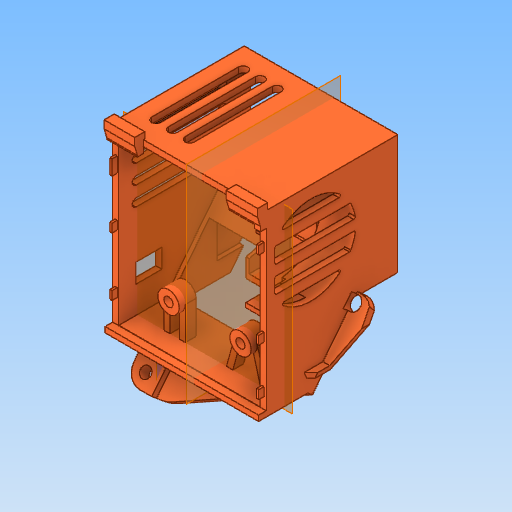
# Autodesk Inventor part: кожух2
Saved by Autodesk Inventor 2017 (Build 210142000, 142)
## iProperties
Part Number: кожух2
Material: Типовые
Document SubType Name: Modeling
Designer: Max
Mass: 19.7684 g
Surface Area: 231.932 cm^2
Volume: 19.7684 cm^3
Density: 1 g/cm^3
Appearance: Оранжевый
Author: Max
Autodesk Inventor part; units mm, degrees
ref_plane "YZ Plane" through (0, 0, 0) normal (1, 0, 0) x (0, 1, 0)
ref_plane "XZ Plane" through (0, 0, 0) normal (0, 1, 0) x (-1, 0, 0)
ref_plane "XY Plane" through (0, 0, 0) normal (0, 0, 1) x (1, 0, 0)
sketch "Эскиз1" plane through (0, 0, 0) normal (0, 0, 1) x (1, 0, 0)
  line L0 (1.3628, -26.8991) -> (1.3628, -29.3491) projected
  line L1 (1.3628, -29.3491) -> (24.1628, -29.3491) projected
  line L2 (24.1628, -29.3491) -> (24.1628, -4.9691) projected
  line L3 (24.1628, -4.9691) -> (13.8628, -4.9691) projected
  line L4 (13.8628, -4.9691) -> (13.8628, 12.3409) projected
  line L5 (13.8628, 12.3409) -> (24.1628, 12.3409) projected
  line L6 (24.1628, 12.3409) -> (24.1628, 22.1409) projected
  line L7 (24.1628, 22.1409) -> (22.1628, 22.1409) projected
  line L8 (22.1628, 22.1409) -> (22.1628, 23.2409) projected
  line L9 (22.1628, 23.2409) -> (19.7628, 23.2409) projected
  line L10 (19.7628, 23.2409) -> (19.7628, 20.2409) projected
  line L11 (19.7628, 20.2409) -> (15.3628, 20.2409) projected
  line L12 (15.3628, 20.2409) -> (15.3628, 23.2409) projected
  line L13 (15.3628, 23.2409) -> (13.8628, 23.2409) projected
  line L14 (13.8628, 23.2409) -> (13.8628, 27.2009) projected
  line L15 (13.8628, 27.2009) -> (-16.0172, 27.2009) projected
  line L16 (-16.0172, 27.2009) -> (-16.0172, 23.2409) projected
  line L17 (-16.0172, 23.2409) -> (-17.1172, 23.2409) projected
  line L18 (-17.1172, 23.2409) -> (-17.1172, 20.2009) projected
  line L19 (-17.1172, 20.2009) -> (-21.5172, 20.2009) projected
  line L20 (-21.5172, 20.2009) -> (-21.5172, 23.2409) projected
  line L21 (-21.5172, 23.2409) -> (-26.0172, 23.2409) projected
  line L22 (-26.0172, 23.2409) -> (-26.0172, -29.3491) projected
  line L23 (-26.0172, -29.3491) -> (-3.1372, -29.3491) projected
  line L24 (-3.1372, -29.3491) -> (-3.1372, -26.8991) projected
  line L25 (-3.1372, -26.8991) -> (1.3628, -26.8991) projected
  line L26 (-6.6027, 20.9009) -> (-7.4672, 20.9009) projected
  arc A0 (-6.6027, 20.9009) -> (-7.2289, 20.2627) centre (-4.7984, 18.5041) ccw projected
  line L27 (-7.2289, 20.2627) -> (-8.0672, 19.1042) projected
  arc A1 (-5.6572, 17.7284) -> (-8.0672, 19.1042) centre (-12.3972, 8.7209) ccw projected
  line L28 (-5.6572, 17.7284) -> (0.0428, 23.0709) projected
  line L29 (0.0428, 23.0709) -> (1.0428, 23.0709) projected
  line L30 (1.0428, 23.0709) -> (1.0428, -5.6291) projected
  line L31 (1.0428, -5.6291) -> (0.0428, -5.6291) projected
  line L32 (0.0428, -5.6291) -> (-3.9933, -1.8461) projected
  arc A2 (-3.9933, -1.8461) -> (-7.3822, -1.3495) centre (-6.0449, -4.0349) ccw projected
  arc A3 (-14.1715, 19.8301) -> (-7.3822, -1.3495) centre (-12.3972, 8.7209) ccw projected
  line L33 (-14.1715, 19.8301) -> (-7.4672, 20.9009) projected
  line L34 (3.2328, 20.0509) -> (3.2328, 26.3009) projected
  line L35 (3.2328, 26.3009) -> (11.7328, 26.3009) projected
  line L36 (11.7328, 26.3009) -> (11.7328, 20.0509) projected
  line L37 (11.7328, 20.0509) -> (3.2328, 20.0509) projected
  line L38 (2.9428, -9.0491) -> (2.9428, -2.8491) projected
  line L39 (2.9428, -2.8491) -> (11.3928, -2.8491) projected
  line L40 (11.3928, -2.8491) -> (11.3928, -9.0491) projected
  line L41 (11.3928, -9.0491) -> (2.9428, -9.0491) projected
  line L42 (11.1828, 15.3909) -> (11.1828, 4.1309) projected
  line L43 (11.1828, 4.1309) -> (3.5128, 4.1309) projected
  line L44 (3.5128, 4.1309) -> (3.5128, 15.3909) projected
  line L45 (3.5128, 15.3909) -> (5.2778, 15.3909) projected
  line L46 (5.2778, 15.3909) -> (5.2778, 7.1309) projected
  line L47 (5.2778, 7.1309) -> (9.4178, 7.1309) projected
  line L48 (9.4178, 7.1309) -> (9.4178, 15.3909) projected
  line L49 (9.4178, 15.3909) -> (11.1828, 15.3909) projected
  line L50 (-16.0372, -26.1691) -> (-16.0372, -22.6691) projected
  line L51 (-16.0372, -22.6691) -> (-10.7672, -22.6691) projected
  line L52 (-10.7672, -22.6691) -> (-10.7672, -26.1691) projected
  line L53 (-10.7672, -26.1691) -> (-16.0372, -26.1691) projected
  line L54 (-21.1172, -9.1491) -> (-21.1172, -6.5491) projected
  line L55 (-21.1172, -6.5491) -> (-15.8172, -6.5491) projected
  line L56 (-15.8172, -6.5491) -> (-15.8172, -9.1491) projected
  line L57 (-15.8172, -9.1491) -> (-21.1172, -9.1491) projected
  circle A4 centre (16.8328, -11.1491) radius 2.05 projected
  circle A5 centre (-11.7672, -18.4991) radius 2.05 projected
  circle A6 centre (11.7328, -18.4991) radius 2.05 projected
  circle A7 centre (-1.1672, -11.1291) radius 1.9 projected
  circle A8 centre (17.9828, 16.4009) radius 1.15 projected
  line L58 (-25.2172, 13.4509) -> (-25.2172, 18.3509) projected
  line L59 (-25.2172, 18.3509) -> (-24.5172, 18.3509) projected
  line L60 (-24.5172, 18.3509) -> (-24.5172, 13.4509) projected
  line L61 (-24.5172, 13.4509) -> (-25.2172, 13.4509) projected
  line L62 (-25.2172, -2.6491) -> (-25.2172, 0.1509) projected
  line L63 (-25.2172, 0.1509) -> (-24.5172, 0.1509) projected
  line L64 (-24.5172, 0.1509) -> (-24.5172, -2.6491) projected
  line L65 (-24.5172, -2.6491) -> (-25.2172, -2.6491) projected
  line L66 (-25.2172, -21.7291) -> (-25.2172, -18.9291) projected
  line L67 (-25.2172, -18.9291) -> (-24.5172, -18.9291) projected
  line L68 (-24.5172, -18.9291) -> (-24.5172, -21.7291) projected
  line L69 (-24.5172, -21.7291) -> (-25.2172, -21.7291) projected
  line L70 (22.7628, 15.1009) -> (22.7628, 17.9009) projected
  line L71 (22.7628, 17.9009) -> (23.4628, 17.9009) projected
  line L72 (23.4628, 17.9009) -> (23.4628, 15.1009) projected
  line L73 (23.4628, 15.1009) -> (22.7628, 15.1009) projected
  line L74 (22.7628, -25.7691) -> (22.7628, -22.9691) projected
  line L75 (22.7628, -22.9691) -> (23.4628, -22.9691) projected
  line L76 (23.4628, -22.9691) -> (23.4628, -25.7691) projected
  line L77 (23.4628, -25.7691) -> (22.7628, -25.7691) projected
  line L78 (22.7628, -10.3691) -> (22.7628, -7.5691) projected
  line L79 (22.7628, -7.5691) -> (23.4628, -7.5691) projected
  line L80 (23.4628, -7.5691) -> (23.4628, -10.3691) projected
  line L81 (23.4628, -10.3691) -> (22.7628, -10.3691) projected
  line L82 (-26.0172, -31.2191) -> (24.1628, -31.2191)
  line L83 (24.1628, -31.2191) -> (24.1628, 27.2009)
  line L84 (24.1628, 27.2009) -> (-26.0172, 27.2009)
  line L85 (-26.0172, 29.2009) -> (-26.0172, -31.2191)
  line L86 (-26.0172, -29.3491) -> (24.1628, -29.3491)
  line L87 (-24.0172, -29.3491) -> (-24.0172, 23.2409)
  line L88 (22.1628, -29.3491) -> (22.1628, 23.2409)
  line L89 (-16.0172, 23.2409) -> (-26.0172, 23.2409)
  line L90 (-26.0172, 29.2009) -> (-16.0172, 29.2009)
  line L91 (-16.0172, 29.2009) -> (-16.0172, 23.2409)
  line L92 (13.8628, 23.2409) -> (22.1628, 23.2409)
  line L93 (24.1628, 23.2409) -> (24.1628, 29.2009)
  line L94 (24.1628, 29.2009) -> (13.8628, 29.2009)
  line L95 (13.8628, 29.2009) -> (13.8628, 23.2409)
  line L96 (22.1628, 22.1409) -> (24.1628, 22.1409)
  line L97 (-26.0172, 23.2409) -> (-26.0172, 29.2009)
  line L98 (-26.0172, -31.2191) -> (24.1628, -31.2191)
  line L99 (24.1628, -31.2191) -> (24.1628, -29.3491)
  line L100 (24.1628, -29.3491) -> (-26.0172, -29.3491)
  line L101 (-26.0172, -29.3491) -> (-26.0172, -31.2191)
  line L102 (22.1628, 22.1409) -> (24.1628, 22.1409)
  line L103 (24.1628, 22.1409) -> (24.1628, -29.3491)
  line L104 (24.1628, -29.3491) -> (22.1628, -29.3491)
  line L105 (22.1628, -29.3491) -> (22.1628, 22.1409)
  line L106 (-24.0172, 23.2409) -> (-26.0172, 23.2409)
  line L107 (-26.0172, 23.2409) -> (-26.0172, -29.3491)
  line L108 (-26.0172, -29.3491) -> (-24.0172, -29.3491)
  line L109 (-24.0172, -29.3491) -> (-24.0172, 23.2409)
  line L110 (-16.0172, 27.2009) -> (13.8628, 27.2009)
  line L111 (13.8628, 27.2009) -> (13.8628, 25.2009)
  line L112 (24.1628, 25.2009) -> (-26.0172, 25.2009)
  line L113 (-16.0172, 25.2009) -> (-16.0172, 27.2009)
  line L114 (24.1628, 25.2009) -> (13.8628, 25.2009)
  line L115 (13.8628, 25.2009) -> (13.8628, 27.2009)
  line L116 (13.8628, 27.2009) -> (24.1628, 27.2009)
  line L117 (24.1628, 27.2009) -> (24.1628, 25.2009)
  line L118 (-26.0172, 25.2009) -> (-16.0172, 25.2009)
  line L119 (-16.0172, 25.2009) -> (-16.0172, 27.2009)
  line L120 (-16.0172, 27.2009) -> (-26.0172, 27.2009)
  line L121 (-26.0172, 27.2009) -> (-26.0172, 25.2009)
  line L122 (-24.0172, 23.2409) -> (-26.0172, 23.2409)
  line L123 (-26.0172, 23.2409) -> (-26.0172, 25.2009)
  line L124 (-26.0172, 25.2009) -> (-24.0172, 25.2009)
  line L125 (-24.0172, 25.2009) -> (-24.0172, 23.2409)
  line L126 (22.1628, 22.1409) -> (24.1628, 22.1409)
  line L127 (24.1628, 22.1409) -> (24.1628, 25.2009)
  line L128 (24.1628, 25.2009) -> (22.1628, 25.2009)
  line L129 (22.1628, 25.2009) -> (22.1628, 22.1409)
  point P0 (0, 0)
  dimension "d0" = 1.87
  dimension "d1" = 2
  dimension "d2" = 2
  dimension "d3" = 2
  dimension "d6" = 2
  constraints: 96 end point, 22 parallel, 13 point on line, 11 horizontal, 11 perpendicular, 7 collinear, 1 vertical
  measures "d0" distance between parallel lines of L23 L82
  measures "d1" distance between parallel lines of L87 L22
  measures "d2" distance between parallel lines of L83 L88
  measures "d3" distance between parallel lines of L15 L90
  measures "d6" distance between parallel lines of L15 L112
extrude "Выдавливание1" add sketch "Эскиз1" against normal blind 43 contours L1 L83 L82 L85 L23 L86 | L88 L3 L2 L1 | L88 L5 L83 L3 | L23 L22 L21 L87 | L88 L7 L6 L5 | L21 L85 L112 L125 | L8 L129 L112 L83 L7 | L112 L85 L84 L16 | L16 L15 L14 L112 L36 L35 L34 | L112 L14 L84 L83 | L85 L90 L91 L84 | L34 L35 L36 L112 | L58 L59 L60 L61 | L62 L63 L64 L65 | L66 L67 L68 L69 | L70 L71 L72 L73 | L74 L75 L76 L77 | L78 L79 L80 L81
extrude "Выдавливание2" cut sketch "Эскиз1" against normal blind 43 contours L85 L90 L91 L84
sketch "Эскиз2" plane through (0, 0, 0) normal (0, 0, 1) x (1, 0, 0)
  line L0 (-16.0172, 29.2009) -> (-16.0172, 23.2409) projected
  line L1 (-26.0172, 29.2009) -> (-16.0172, 29.2009) projected
  line L2 (-16.0172, 23.2409) -> (-26.0172, 23.2409) projected
  line L3 (13.8628, 23.2409) -> (13.8628, 27.2009) projected
  line L4 (13.8628, 29.2009) -> (13.8628, 23.2409) projected
  line L5 (24.1628, 29.2009) -> (13.8628, 29.2009) projected
  line L6 (24.1628, 23.2409) -> (24.1628, 29.2009) projected
  line L7 (24.1628, 22.1409) -> (22.1628, 22.1409) projected
  line L8 (22.1628, 25.2009) -> (22.1628, -29.3491) projected
  line L9 (22.1628, 23.2409) -> (19.7628, 23.2409) projected
  line L10 (13.8628, 23.2409) -> (22.1628, 23.2409) projected
  line L11 (24.1628, 23.2409) -> (24.1628, 22.1409)
  line L12 (24.1628, -31.2191) -> (24.1628, 27.2009) projected
  line L13 (-26.0172, 23.2409) -> (-26.0172, 29.2009)
  line L14 (-26.0172, -31.2191) -> (-26.0172, 27.2009) projected
  point P0 (0, 0)
  constraints: 4 end point, 2 collinear
extrude "Выдавливание3" add sketch "Эскиз2" along normal blind 2.8
sketch "Эскиз3" plane through (24.1628, -31.2191, -43) normal (1, 0, 0) x (0, 0, -1)
  line L0 (-43, 53.36) -> (-45.8, 53.36) projected
  line L1 (-44.92, 53.36) -> (-44.92, 54.8992)
  line L2 (-44.92, 54.8992) -> (-45.8, 57.8704)
  line L3 (-45.8, 53.36) -> (-45.8, 60.42) projected
  line L4 (-45.8, 54.46) -> (-45.8, 53.36) projected
  line L5 (-45.8, 57.8704) -> (-45.8, 53.36)
  line L6 (-44.92, 53.36) -> (-45.8, 53.36)
  point P0 (-43, 31.2191)
  dimension "d11" = 1.92
  constraints: 8 end point, 2 collinear, 2 point on line, 1 vertical
  measures "d11" distance from line of L0.start L1
extrude "Выдавливание4" cut sketch "Эскиз3" against normal blind 55
extrude "Выдавливание5" add sketch "Эскиз1" along normal blind 1.73 contours L58 L59 L60 L61 | L62 L63 L64 L65 | L66 L67 L68 L69 | L70 L71 L72 L73 | L74 L75 L76 L77 | L78 L79 L80 L81
sketch "Эскиз4" plane through (0, 0, 0) normal (0, 0, 1) x (1, 0, 0)
  line L0 (-26.0172, -31.2191) -> (24.1628, -31.2191) projected
  line L1 (-26.0172, -31.2191) -> (24.1628, -31.2191)
  line L2 (24.1628, -31.2191) -> (24.1628, -29.4423)
  line L3 (24.1628, -29.4423) -> (-26.0172, -29.4423)
  line L4 (-26.0172, -29.4423) -> (-26.0172, -31.2191)
  point P0 (0, 0)
  constraints: 8 end point, 2 parallel, 1 horizontal, 1 perpendicular
extrude "Выдавливание6" add sketch "Эскиз4" along normal blind 2.5
sketch "Эскиз5" plane through (24.1628, -31.2191, -43) normal (1, 0, 0) x (0, 0, -1)
  arc A0 (-42.5564, 43.56) -> (-25.7, 25.4421) centre (-28.25, 39.97) ccw projected
  arc A1 (-25.7, 54.4979) -> (-41, 47.3862) centre (-28.25, 39.97) ccw projected
  arc A2 (-37.57, 28.862) -> (-18.93, 28.862) centre (-28.25, 39.97) ccw
  line L0 (-43, 58.42) -> (0, 58.42) projected
  line L1 (-43, 1.7768) -> (-43, 53.36) projected
  line L2 (-28.25, 39.97) -> (-36.4963, 39.97) construction
  line L3 (-39.7, 38.295) -> (-14.42, 38.295)
  line L4 (-14.42, 41.645) -> (-39.7, 41.645)
  line L5 (-37.2486, 29.745) -> (-19.2514, 29.745)
  line L6 (-39.7, 46.845) -> (-15.7857, 46.845)
  line L7 (-19.2514, 50.195) -> (-37.2486, 50.195)
  line L8 (-15.7857, 33.095) -> (-39.7, 33.095)
  arc A3 (-37.2486, 29.745) -> (-37.57, 28.862) centre (-37.2486, 29.245) ccw
  arc A4 (-18.93, 28.862) -> (-19.2514, 29.745) centre (-19.2514, 29.245) ccw
  arc A5 (-18.93, 51.078) -> (-37.57, 51.078) centre (-28.25, 39.97) ccw
  arc A6 (-15.3405, 33.3673) -> (-13.9261, 37.7173) centre (-28.25, 39.97) ccw
  arc A7 (-13.9261, 42.2227) -> (-15.3405, 46.5727) centre (-28.25, 39.97) ccw
  line L9 (-40.2, 33.595) -> (-40.2, 37.795)
  line L10 (-40.2, 42.145) -> (-40.2, 46.345)
  arc A8 (-37.57, 51.078) -> (-37.2486, 50.195) centre (-37.2486, 50.695) ccw
  arc A9 (-19.2514, 50.195) -> (-18.93, 51.078) centre (-19.2514, 50.695) ccw
  arc A10 (-15.3405, 46.5727) -> (-15.7857, 46.845) centre (-15.7857, 46.345) ccw
  arc A11 (-14.42, 41.645) -> (-13.9261, 42.2227) centre (-14.42, 42.145) ccw
  arc A12 (-13.9261, 37.7173) -> (-14.42, 38.295) centre (-14.42, 37.795) ccw
  arc A13 (-15.7857, 33.095) -> (-15.3405, 33.3673) centre (-15.7857, 33.595) ccw
  arc A14 (-40.2, 33.595) -> (-39.7, 33.095) centre (-39.7, 33.595) ccw
  arc A15 (-39.7, 38.295) -> (-40.2, 37.795) centre (-39.7, 37.795) ccw
  arc A16 (-40.2, 42.145) -> (-39.7, 41.645) centre (-39.7, 42.145) ccw
  arc A17 (-39.7, 46.845) -> (-40.2, 46.345) centre (-39.7, 46.345) ccw
  point P0 (-43, 31.2191)
  point P1 (-13.8471, 38.295)
  point P2 (-13.8471, 41.645)
  point P3 (-15.4835, 33.095)
  point P4 (-38.531, 29.745)
  point P5 (-17.969, 29.745)
  point P6 (-15.4835, 46.845)
  point P7 (-17.969, 50.195)
  point P8 (-38.531, 50.195)
  dimension "d18" = 29
  dimension "d21" = 3.35
  dimension "d23" = 3.35
  dimension "d25" = 5.2
  dimension "d26" = 3.35
  dimension "d27" = 5.2
  dimension "d28" = 0.5
  dimension "d29" = 2.8
  dimension "d30" = 2.8
  dimension "d31" = 0.5
  constraints: 36 point on circle, 22 tangent, 18 end point, 15 centre point, 10 equal radius, 8 point on line, 4 coincident, 4 horizontal, 3 parallel, 2 vertical, 16 other
  measures "d21" distance between parallel lines of L4 L3
  measures "d23" distance between parallel lines of L7 L6
  measures "d25" distance between parallel lines of L4 L6
  measures "d26" distance between parallel lines of L5 L8
  measures "d27" distance between parallel lines of L3 L8
  measures "d28" radius of A3
  measures "d29" distance between parallel lines of L1 L10
  measures "d30" distance between parallel lines of L1 L9
  measures "d31" radius of A8
extrude "Выдавливание7" cut sketch "Эскиз5" against normal blind 2.5
sketch "Эскиз7" plane through (24.1628, -31.2191, -43) normal (1, 0, 0) x (0, 0, -1)
  arc A0 (-37.57, 28.862) -> (-18.93, 28.862) centre (-28.25, 39.97) ccw projected
  arc A1 (-37.57, 28.862) -> (-18.93, 28.862) centre (-28.25, 39.97) ccw projected
  circle A2 centre (-28.25, 39.97) radius 14.5
  line L0 (-28.25, 23.97) -> (-39.4, 23.97)
  line L1 (-39.4, 23.97) -> (-39.4, 25.47)
  line L2 (-39.4, 25.47) -> (-28.25, 25.47)
  arc A3 (-18.93, 51.078) -> (-37.57, 51.078) centre (-28.25, 39.97) ccw projected
  line L3 (-28.25, 54.47) -> (-44.92, 54.47)
  line L4 (-43, 53.36) -> (-44.92, 53.36) projected
  line L5 (-44.92, 54.46) -> (-44.92, 54.8992) projected
  line L6 (-44.92, 54.47) -> (-44.92, 54.8992)
  line L7 (-45.8, 57.8704) -> (-44.92, 54.8992) projected
  line L8 (-44.92, 54.8992) -> (-45.8, 57.8704)
  line L9 (-43, 60.42) -> (-45.8, 60.42) projected
  line L10 (-45.8, 57.8704) -> (-45.8, 60.42)
  line L11 (-45.8, 60.42) -> (-43, 60.42)
  line L12 (-43, 58.42) -> (-43, 60.42) projected
  line L13 (-43, 58.42) -> (-43, 60.42)
  line L14 (-43, 60.42) -> (-43, 58.42)
  line L15 (-43, 58.42) -> (-12.3, 58.42)
  line L16 (-43, 58.42) -> (0, 58.42) projected
  line L17 (-12.3, 58.42) -> (-12.3, 54.47)
  line L18 (-12.3, 54.47) -> (-28.25, 54.47)
  line L19 (0, 58.42) -> (0, 0) projected
  arc A4 (-28.25, 23.97) -> (-21.4861, 54.47) centre (-28.25, 39.97) ccw
  line L20 (-43, 1.7768) -> (-43, 53.36) projected
  point P0 (-43, 31.2191)
  dimension "d35" = 12.3
  dimension "d36" = 1.5
  dimension "d37" = 3.6
  constraints: 26 end point, 6 point on circle, 5 collinear, 3 perpendicular, 3 point on line, 2 centre point, 2 coincident, 2 parallel, 2 tangent, 1 horizontal
  measures "d35" distance between parallel lines of L19 L17
  measures "d36" distance between parallel lines of L2 L0
  measures "d37" distance between parallel lines of L1 L20
extrude "Выдавливание8" add sketch "Эскиз7" against normal up to surface (10.3 mm away) contours A0 A2 L18 A4 L0 L1 L2 | L3 L5 L7 L10 L9 L12 L15 L17 L18
sketch "Эскиз9" plane through (0, 0, -43) normal (0, 0, -1) x (-1, 0, 0)
  line L0 (26.0172, 27.2009) -> (-24.1628, 27.2009) projected
  line L1 (-24.1628, 27.2009) -> (-24.1628, -31.2191) projected
  line L2 (-24.1628, -31.2191) -> (26.0172, -31.2191) projected
  line L3 (26.0172, -31.2191) -> (26.0172, 27.2009) projected
  line L4 (-22.1628, 25.2009) -> (24.0172, 25.2009) projected
  line L5 (24.0172, 25.2009) -> (24.0172, -29.3491) projected
  line L6 (24.0172, -29.3491) -> (-22.1628, -29.3491) projected
  line L7 (-22.1628, -29.3491) -> (-22.1628, 25.2009) projected
  line L8 (-24.1628, -29.4423) -> (-24.1628, 22.1409) projected
  line L9 (-24.1628, -11.7991) -> (0.9972, -11.7991)
  line L10 (0.9972, -11.7991) -> (0.9972, -9.9991)
  line L11 (0.9972, -9.9991) -> (-24.1628, -9.9991)
  line L12 (-24.1628, -9.9991) -> (-24.1628, -11.7991)
  line L13 (0.9972, -11.7991) -> (2.8372, -11.7991)
  line L14 (2.8372, -11.7991) -> (2.8372, 1.6982)
  line L15 (2.8372, 1.6982) -> (0.9972, 1.6982)
  line L16 (0.9972, 1.6982) -> (0.9972, -11.7991)
  line L17 (0.1387, -9.9991) -> (-22.1628, -9.9991)
  line L18 (-22.1628, -9.9991) -> (-22.1628, 25.2009)
  line L19 (-22.1628, 25.2009) -> (0.1387, 25.2009)
  line L20 (0.1387, 25.2009) -> (0.1387, -9.9991)
  line L21 (2.8372, -11.7991) -> (0.9972, -11.7991)
  line L22 (0.9972, -11.7991) -> (0.9972, -19.2291)
  line L23 (0.9972, -19.2291) -> (2.8372, -19.2291)
  line L24 (2.8372, -19.2291) -> (2.8372, -11.7991)
  point P0 (0, 0)
  dimension "d42" = 23.16
  dimension "d43" = 1.84
  dimension "d44" = 1.8
  dimension "d45" = 7.43
  dimension "d46" = 35.2
  constraints: 32 end point, 8 parallel, 4 horizontal, 4 perpendicular, 2 point on line, 1 collinear
  measures "d42" distance between parallel lines of L7 L16
  measures "d43" distance between parallel lines of L16 L14
  measures "d44" distance between parallel lines of L11 L9
  measures "d45" distance between parallel lines of L9 L23
  measures "d46" distance between parallel lines of L19 L17
extrude "Выдавливание9" add sketch "Эскиз9" against normal blind 12.3 contours L11 L7 L9 L1 | L11 L10 L9 L7 | L10 L16 L15 L14 L13 | L13 L24 L23 L22
sketch "Эскиз10" plane through (22.1628, 23.2509, -30.7) normal (0, 0, -1) x (-1, 0, 0)
  line L0 (8.3, 0) -> (8.3, 1.95) projected
  line L1 (0, 1.95) -> (46.18, 1.95) projected
  line L2 (8.3, 0) -> (21.1, 0)
  line L3 (21.1, 0) -> (21.1, 1.95)
  line L4 (21.1, 1.95) -> (8.3, 1.95)
  line L5 (8.3, 1.95) -> (8.3, 0)
  line L6 (21.1, 0) -> (8.3, 0)
  line L7 (8.3, 0) -> (8.3, -33.25)
  line L8 (8.3, -33.25) -> (21.1, -33.25)
  line L9 (21.1, -33.25) -> (21.1, 0)
  line L10 (8.3, -29) -> (8.3, -30.5) projected
  line L11 (23.16, -33.25) -> (0, -33.25) projected
  line L12 (18.67, -28.55) -> (10.73, -28.55)
  line L13 (10.73, -28.55) -> (10.73, -20.35)
  line L14 (10.73, -20.35) -> (18.67, -20.35)
  line L15 (18.67, -20.35) -> (18.67, -28.55)
  line L16 (18.67, -9.6) -> (10.73, -9.6)
  line L17 (10.73, -9.6) -> (10.73, -1.4)
  line L18 (10.73, -1.4) -> (18.67, -1.4)
  line L19 (18.67, -1.4) -> (18.67, -9.6)
  line L20 (48.18, 3.95) -> (-2, 3.95) projected
  line L21 (0, -35.05) -> (23.16, -35.05) projected
  line L22 (17.87, -20.35) -> (11.53, -20.35)
  line L23 (11.53, -20.35) -> (11.53, -27.75)
  line L24 (11.53, -27.75) -> (17.87, -27.75)
  line L25 (17.87, -27.75) -> (17.87, -20.35)
  line L26 (17.87, -1.4) -> (11.53, -1.4)
  line L27 (11.53, -2.2) -> (11.53, -9.6)
  line L28 (17.87, -9.6) -> (17.87, -2.2)
  line L29 (17.87, -2.2) -> (11.53, -2.2)
  point P0 (22.1628, -23.2509)
  dimension "d49" = 12.8
  dimension "d50" = 2.43
  dimension "d51" = 2.43
  dimension "d52" = 5.35
  dimension "d53" = 1.4
  dimension "d54" = 6.5
  dimension "d55" = 8.2
  dimension "d56" = 8.2
  dimension "d57" = 0.8
  dimension "d58" = 0.8
  dimension "d59" = 0.8
  dimension "d60" = 0.8
  constraints: 48 end point, 11 parallel, 8 point on line, 7 perpendicular, 6 horizontal, 4 collinear
  measures "d49" distance between parallel lines of L7 L9
  measures "d50" distance between parallel lines of L9 L15
  measures "d51" distance between parallel lines of L7 L13
  measures "d52" distance between parallel lines of L18 L20
  measures "d53" distance between parallel lines of L18 L2
  measures "d54" distance between parallel lines of L12 L21
  measures "d55" distance between parallel lines of L18 L16
  measures "d56" distance between parallel lines of L14 L12
  measures "d57" distance between parallel lines of L15 L25
  measures "d58" distance between parallel lines of L13 L23
  measures "d59" distance between parallel lines of L12 L24
  measures "d60" distance between parallel lines of L18 L29
extrude "Выдавливание10" add sketch "Эскиз10" against normal blind 0.8 contours L0 L1 L3 L2 | L2 L9 L8 L7 | L25 L24 L23 L14 | L16 L27 L29 L28
sketch "Эскиз11" plane through (22.1628, 23.2509, -29.9) normal (0, 0, 1) x (1, 0, 0)
  line L0 (-18.67, -20.35) -> (-17.87, -20.35) projected
  line L1 (-17.87, -20.35) -> (-17.87, -27.75) projected
  line L2 (-17.87, -27.75) -> (-11.53, -27.75) projected
  line L3 (-11.53, -27.75) -> (-11.53, -20.35) projected
  line L4 (-11.53, -20.35) -> (-10.73, -20.35) projected
  line L5 (-10.73, -20.35) -> (-10.73, -28.55) projected
  line L6 (-10.73, -28.55) -> (-18.67, -28.55) projected
  line L7 (-18.67, -28.55) -> (-18.67, -20.35) projected
  line L8 (-18.67, -1.4) -> (-10.73, -1.4) projected
  line L9 (-10.73, -1.4) -> (-10.73, -9.6) projected
  line L10 (-10.73, -9.6) -> (-11.53, -9.6) projected
  line L11 (-11.53, -9.6) -> (-11.53, -2.2) projected
  line L12 (-11.53, -2.2) -> (-17.87, -2.2) projected
  line L13 (-17.87, -2.2) -> (-17.87, -9.6) projected
  line L14 (-17.87, -9.6) -> (-18.67, -9.6) projected
  line L15 (-18.67, -9.6) -> (-18.67, -1.4) projected
  line L16 (-8.3, -33.25) -> (-8.3, -19.6456) projected
  line L17 (-8.3, -9.3544) -> (-8.3, -19.6456) projected
  line L18 (-8.3, -9.3544) -> (-8.3, 0) projected
  line L19 (-8.3, 1.95) -> (-8.3, 0) projected
  line L20 (-21.1, 1.95) -> (-8.3, 1.95) projected
  line L21 (-21.1, 1.95) -> (-21.1, -33.25) projected
  line L22 (-21.1, -33.25) -> (-8.3, -33.25) construction
  line L23 (0, -33.25) -> (0, -35.05) projected
  line L24 (-21.1, -33.25) -> (-8.3, -33.25) projected
  line L25 (-21.1, -33.25) -> (-23.16, -33.25) projected
  line L26 (-23.16, -33.25) -> (-23.16, -21.5527) projected
  line L27 (-23.16, -21.5527) -> (-25, -21.5527) projected
  line L28 (-25, -21.5527) -> (-25, -42.48) projected
  line L29 (-25, -42.48) -> (-23.16, -42.48) projected
  line L30 (-23.16, -42.48) -> (-23.16, -35.05) projected
  line L31 (-23.16, -35.05) -> (0, -35.05) construction
  line L32 (-23.16, -35.05) -> (0, -35.05) projected
  line L33 (-21.1, -33.25) -> (-21.1, 1.95) projected
  line L34 (-8.3, -35.05) -> (-21.1, -35.05)
  line L35 (-21.1, -35.05) -> (-21.1, 1.95)
  line L36 (-21.1, 1.95) -> (-8.3, 1.95)
  line L37 (-8.3, 1.95) -> (-8.3, -35.05)
  line L38 (-9.3, 0.95) -> (-20.1, 0.95)
  line L39 (-20.1, 0.95) -> (-20.1, -33.25)
  line L40 (-20.1, -33.25) -> (-9.3, -33.25)
  line L41 (-9.3, -33.25) -> (-9.3, 0.95)
  point P0 (-22.1628, -23.2509)
  dimension "d63" = 1
  dimension "d64" = 1
  dimension "d65" = 1
  constraints: 16 end point, 4 parallel, 2 horizontal, 2 perpendicular, 1 collinear, 1 point on line
  measures "d63" distance between parallel lines of L20 L38
  measures "d64" distance between parallel lines of L33 L39
  measures "d65" distance between parallel lines of L17 L41
extrude "Выдавливание11" add sketch "Эскиз11" along normal blind 13.4 contours L24 L41 L38 L39 L21 L20 L19 L18 L17 L16 | L37 L32 L35 L24
sketch "Эскиз12" plane through (22.1628, 23.2509, -29.9) normal (0, 0, -1) x (-1, 0, 0)
  line L0 (21.1, -33.25) -> (20.1, -33.25) projected
  line L1 (20.1, -33.25) -> (9.3, -33.25) projected
  line L2 (9.3, -33.25) -> (8.3, -33.25) projected
  line L3 (8.3, -35.05) -> (8.3, -33.25) projected
  line L4 (21.1, -35.05) -> (8.3, -35.05) projected
  line L5 (21.1, -33.25) -> (21.1, -35.05) projected
  point P0 (22.1628, -23.2509)
extrude "Выдавливание12" add sketch "Эскиз12" along normal blind 1
sketch "Эскиз13" plane through (12.8628, -9.9991, -29.9) normal (-1, 0, 0) x (0, 0, 1)
  arc A0 (15.15, 4.25) -> (24.47, 7.642) centre (15.15, 18.75) ccw projected
  circle A1 centre (15.15, 18.75) radius 14.5
  point P0 (29.9, 9.9991)
  dimension "d70" = 29
  constraints: 1 centre point, 1 coincident
  measures "d70" diameter of A1
extrude "Выдавливание13" cut sketch "Эскиз13" along normal blind 15 and the other way blind 3
sketch "Эскиз14" plane through (22.1628, 23.2509, -30.7) normal (0, 0, -1) x (-1, 0, 0)
  line L0 (8.3, -0.01) -> (0, -0.01) projected
  line L1 (0, -0.01) -> (6, -0.01)
  line L2 (6, -0.01) -> (6, -5.01)
  line L3 (6, -5.01) -> (0, -5.01)
  line L4 (0, -5.01) -> (0, -0.01)
  point P0 (22.1628, -23.2509)
  dimension "d75" = 6
  dimension "d76" = 5
  constraints: 8 end point, 2 parallel, 1 horizontal, 1 perpendicular
  measures "d75" distance between parallel lines of L4 L2
  measures "d76" distance between parallel lines of L0 L3
extrude "Выдавливание14" cut sketch "Эскиз14" against normal blind 15
sketch "Эскиз15" plane through (22.1628, -29.3491, -43) normal (-1, 0, 0) x (0, 0, 1)
  line L0 (39.7, 44.975) -> (15.7857, 44.975) projected
  line L1 (39.4, 44.975) -> (14.6689, 44.975)
  line L2 (14.6689, 44.975) -> (14.6689, 45.855)
  line L3 (14.6689, 45.855) -> (39.4, 45.855)
  line L4 (39.4, 45.855) -> (39.4, 44.975)
  line L5 (43, -0.0932) -> (43, 51.49) projected
  point P0 (43, 29.3491)
  dimension "d79" = 0.88
  dimension "d80" = 3.6
  constraints: 8 end point, 2 parallel, 1 horizontal, 1 perpendicular, 1 point on line
  measures "d79" distance between parallel lines of L0 L3
  measures "d80" distance between parallel lines of L4 L5
extrude "Выдавливание15" add sketch "Эскиз15" along normal blind 5
sketch "Эскиз16" plane through (-0.9972, -19.2291, -43) normal (1, 0, 0) x (0, 0, -1)
  line L0 (0, 0) -> (-12.3, 0) projected
  line L1 (-1.5, 0) -> (-12.3, 7.43)
  line L2 (-12.3, 20.9273) -> (-12.3, 0) projected
  line L3 (-12.3, 7.43) -> (-12.3, 0)
  line L4 (-1.5, 0) -> (-12.3, 0)
  point P0 (-43, 19.2291)
  dimension "d85" = 7.43
  dimension "d86" = 1.5
  constraints: 6 end point, 2 collinear, 2 point on line
  measures "d85" distance from line of L0 L1.end
  measures "d86" distance of L0.start L1.start
extrude "Выдавливание16" cut sketch "Эскиз16" against normal blind 5
fillet "Сопряжение1" radius 1 2 edges at (-1.9172, -19.2291, -43) (-1.9172, -19.2291, -41.5)
sketch "Эскиз17" plane through (-0.9972, -9.9991, -43) normal (1, 0, 0) x (0, 0, -1)
  line L0 (-3.738, 11.6973) -> (-14.78, -2.4358)
  line L1 (-12.3, 11.6973) -> (-12.3, -1.8) projected
  line L2 (0, 11.6973) -> (-12.3, 11.6973) projected
  line L3 (-3.738, 11.6973) -> (0, 11.6973)
  line L4 (-3.738, 11.6973) -> (-12.3, 11.6973)
  line L5 (-12.3, 11.6973) -> (-12.3, 0.7385)
  line L6 (0, 35.2) -> (0, -19.35) projected
  line L7 (-1.2, 11.6973) -> (-12.242, -2.4358)
  line L8 (-1.2, 11.6973) -> (-3.738, 11.6973)
  line L9 (-12.242, -2.4358) -> (-14.8205, -2.4358)
  point P0 (-43, 9.9991)
  dimension "d90" = 38
  dimension "d91" = 1.2
  dimension "d92" = 2
  dimension "d94" = 19.6
  constraints: 14 end point, 4 point on line, 2 horizontal, 1 collinear, 1 parallel, 1 perpendicular
  measures "d90" angle of L6 L7
  measures "d91" distance from line of L6 L7.start
  measures "d92" distance between parallel lines of L0 L7
  measures "d94" distance of L7.start L0.end
extrude "Выдавливание17" add sketch "Эскиз17" against normal up to surface (23.02 mm away) contours L2 L7 L9 L0
extrude "Выдавливание18" cut sketch "Эскиз17" against normal blind 5 contours L0 L1 L2
sketch "Эскиз19" plane through (24.1628, -31.2191, -43) normal (1, 0, 0) x (0, 0, -1)
  line L0 (0, 19.42) -> (-12.3, 19.42) projected
  line L1 (-1.2, 32.9173) -> (-12.242, 18.7842) projected
  line L2 (-12.242, 18.7842) -> (-33.1562, -7.9848)
  line L3 (-33.1562, -7.9848) -> (6.953, -7.9848)
  line L4 (-3.738, 32.9173) -> (-14.78, 18.7842) projected
  line L5 (-14.78, 18.7842) -> (-12.242, 18.7842) projected
  line L6 (-12.242, 18.7842) -> (-11.9392, 19.1718) projected
  line L7 (-11.9392, 19.1718) -> (-1.756, 12.1661) projected
  arc A0 (-1.756, 12.1661) -> (-1.1892, 11.99) centre (-1.1892, 12.99) ccw projected
  line L8 (-1, 11.99) -> (-1.1892, 11.99) projected
  arc A1 (-1, 11.99) -> (0, 12.99) centre (-1, 12.99) ccw projected
  line L9 (0, 19.42) -> (0, 12.99) projected
  line L10 (0, 19.42) -> (-12.3, 19.42) projected
  line L11 (-12.3, 21.22) -> (-12.3, 19.42) projected
  line L12 (0, 21.22) -> (-12.3, 21.22) projected
  line L13 (0, 32.9173) -> (0, 21.22) projected
  line L14 (0, 32.9173) -> (-3.738, 32.9173) projected
  arc A2 (-1, 11.99) -> (0, 12.99) centre (-1, 12.99) ccw projected
  line L15 (0, 12.99) -> (13.9751, 12.99)
  line L16 (13.9751, 12.99) -> (13.9751, -9.8158)
  line L17 (13.9751, -9.8158) -> (6.953, -7.9848)
  line L18 (-12.242, 18.7842) -> (-11.9392, 19.1718) projected
  line L19 (-12.242, 18.7842) -> (-11.9392, 19.1718)
  line L20 (-11.9392, 19.1718) -> (-1.756, 12.1661) projected
  line L21 (-11.9392, 19.1718) -> (-1.756, 12.1661)
  line L22 (-1.756, 12.1661) -> (-11.9392, 19.1718) projected
  line L23 (-11.9392, 19.1718) -> (-11.7452, 19.42)
  line L24 (-12.3, 19.42) -> (0, 19.42) projected
  line L25 (-11.7452, 19.42) -> (0, 19.42)
  line L26 (0, 56.42) -> (0, 1.87) projected
  line L27 (0, 19.42) -> (0, 12.99)
  point P0 (-43, 31.2191)
  constraints: 20 end point, 2 collinear, 2 horizontal, 2 perpendicular, 2 point on line
extrude "Выдавливание19" cut sketch "Эскиз19" against normal blind 46.8 contours L15 L16 L17 L3 L2 L1 L7 A0 L8 A1
extrude "Выдавливание20" cut sketch "Эскиз19" against normal blind 5 contours L9 A1 L8 A0 L7 L1 L0
sketch "Эскиз20" plane through (24.1628, 27.2009, 0) normal (1, 0, 0) x (0, 0, -1)
  arc A0 (5.43, -29.558) -> (24.07, -29.558) centre (14.75, -18.45) ccw projected
  arc A1 (5.7514, -28.675) -> (5.43, -29.558) centre (5.7514, -29.175) ccw projected
  line L0 (5.7514, -28.675) -> (23.7486, -28.675) projected
  arc A2 (24.07, -29.558) -> (23.7486, -28.675) centre (23.7486, -29.175) ccw projected
  arc A3 (23.7486, -8.225) -> (24.07, -7.342) centre (23.7486, -7.725) ccw projected
  line L1 (23.7486, -8.225) -> (5.7514, -8.225) projected
  arc A4 (5.43, -7.342) -> (5.7514, -8.225) centre (5.7514, -7.725) ccw projected
  arc A5 (24.07, -7.342) -> (5.43, -7.342) centre (14.75, -18.45) ccw projected
  arc A6 (27.6595, -25.0527) -> (29.0739, -20.7027) centre (14.75, -18.45) ccw projected
  arc A7 (27.2143, -25.325) -> (27.6595, -25.0527) centre (27.2143, -24.825) ccw projected
  line L2 (27.2143, -25.325) -> (3.3, -25.325) projected
  arc A8 (2.8, -24.825) -> (3.3, -25.325) centre (3.3, -24.825) ccw projected
  line L3 (2.8, -24.825) -> (2.8, -20.625) projected
  arc A9 (3.3, -20.125) -> (2.8, -20.625) centre (3.3, -20.625) ccw projected
  line L4 (3.3, -20.125) -> (28.58, -20.125) projected
  arc A10 (29.0739, -20.7027) -> (28.58, -20.125) centre (28.58, -20.625) ccw projected
  arc A11 (28.58, -16.775) -> (29.0739, -16.1973) centre (28.58, -16.275) ccw projected
  line L5 (28.58, -16.775) -> (3.3, -16.775) projected
  arc A12 (2.8, -16.275) -> (3.3, -16.775) centre (3.3, -16.275) ccw projected
  line L6 (2.8, -16.275) -> (2.8, -12.075) projected
  arc A13 (3.3, -11.575) -> (2.8, -12.075) centre (3.3, -12.075) ccw projected
  line L7 (3.3, -11.575) -> (27.2143, -11.575) projected
  arc A14 (27.6595, -11.8473) -> (27.2143, -11.575) centre (27.2143, -12.075) ccw projected
  arc A15 (29.0739, -16.1973) -> (27.6595, -11.8473) centre (14.75, -18.45) ccw projected
  line L8 (16.0822, -58.42) -> (31.2548, -39) projected
  line L9 (31.2548, -39) -> (43, -39) projected
  line L10 (43, 0) -> (43, -39) projected
  line L11 (0, 0) -> (43, 0) projected
  line L12 (0, 0) -> (0, 2) projected
  line L13 (0, 2) -> (-2.8, 2) projected
  line L14 (-2.8, -0.5496) -> (-2.8, 2) projected
  line L15 (-2.8, -0.5496) -> (-1.92, -3.5208) projected
  line L16 (-1.92, -3.5208) -> (-1.92, -5.06) projected
  line L17 (0, -5.06) -> (-1.92, -5.06) projected
  line L18 (0, -56.6432) -> (0, -5.06) projected
  line L19 (0, -56.6432) -> (-2.5, -56.6432) projected
  line L20 (-2.5, -58.42) -> (-2.5, -56.6432) projected
  line L21 (16.0822, -58.42) -> (-2.5, -58.42) projected
  line L22 (16.0822, -58.42) -> (31.2548, -39) projected
  line L23 (19.5199, -54.02) -> (12.5199, -54.02)
  line L24 (12.5199, -54.02) -> (12.5199, -52.02)
  line L25 (12.5199, -52.02) -> (18.5444, -52.02)
  line L26 (18.5444, -52.02) -> (29.6932, -37.7502)
  line L27 (29.6932, -37.7502) -> (31.2692, -38.9815)
  line L28 (31.0608, -39.2482) -> (41.8, -25.5027) projected
  line L29 (31.2692, -38.9815) -> (31.2548, -39)
  line L30 (31.2548, -39) -> (17.5432, -56.55) projected
  line L31 (29.3016, -41.5) -> (26.7635, -41.5)
  point P0 (0, -27.2009)
  dimension "d103" = 38
  dimension "d104" = 2
  dimension "d107" = 7
  dimension "d108" = 2
  dimension "d109" = 4.4
  dimension "d110" = 2.5
  constraints: 14 end point, 4 point on line, 3 perpendicular, 2 horizontal, 1 parallel
  measures "d103" angle of L10 L28
  measures "d104" distance between parallel lines of L8 L26
  measures "d107" distance from line of L23.start L24
  measures "d108" distance between parallel lines of L23 L25
  measures "d109" distance between parallel lines of L21 L23
  measures "d110" distance between parallel lines of L9 L31
extrude "Выдавливание21" add sketch "Эскиз20" along normal blind 5.8 contours L23 L24 L25 L26 L31 L8 | L31 L26 L27 L28 L8
extrude "Выдавливание22" add sketch "Эскиз20" against normal up to surface (25.16 mm away) contours L31 L26 L27 L28 L8
fillet "Сопряжение2" radius 10 1 edges at (22.1628, -14.2991, -28.0325)
fillet "Сопряжение3" radius 4 1 edges at (29.9628, -11.165, -30.4812)
sketch "Эскиз21" plane through (0, 0, -43) normal (0, 0, -1) x (-1, 0, 0)
  line L0 (-28.9508, -10.5493) -> (-29.9628, -16.0271)
  line L1 (-29.9628, -26.8191) -> (-29.9628, -14.9327) projected
  line L2 (-29.9628, -16.0271) -> (-25.4506, -27.155)
  line L3 (-25.4506, -27.155) -> (-26.3713, -30.6763)
  line L4 (-26.3713, -30.6763) -> (-32.1863, -30.3048)
  line L5 (-32.1863, -30.3048) -> (-34.0993, -18.0075)
  arc A0 (-33.8339, -17.0111) -> (-34.0993, -18.0075) centre (-32.8346, -17.8108) ccw
  line L6 (-33.8339, -17.0111) -> (-33.212, -11.2122)
  line L7 (-33.212, -11.2122) -> (-28.9508, -10.5493)
  point P0 (0, 0)
  constraints: 14 end point, 2 point on circle, 1 centre point, 1 perpendicular, 1 point on line, 1 tangent
extrude "Выдавливание23" cut sketch "Эскиз21" against normal blind 50
sketch "Эскиз22" plane through (24.1628, -11.7991, -31.2548) normal (0, -0.6156615, -0.7880108) x (-1, 0, 0)
  circle A0 centre (-2.6539, -4.3253) radius 1.75
  point P0 (24.1628, -9.9445)
  dimension "d117" = 3.5
  constraints: 1 centre point
  measures "d117" diameter of A0
extrude "Выдавливание24" cut sketch "Эскиз22" against normal blind 5
sketch "Эскиз23" plane through (-22.6372, -31.2191, -43) normal (1, 0, 0) x (0, 0, -1)
  line L0 (-26.9178, 0) -> (-25.4568, 1.87) projected
  line L1 (-12.242, 18.7842) -> (-25.4568, 1.87)
  line L2 (-12.242, 18.7842) -> (-14.78, 18.7842)
  line L3 (-14.78, 18.7842) -> (-27.9948, 1.87)
  line L4 (0, 1.87) -> (-43, 1.87) projected
  line L5 (-27.9948, 1.87) -> (-25.4568, 1.87)
  line L6 (-12.242, 18.7842) -> (-14.78, 18.7842) projected
  line L7 (-12.242, 18.7842) -> (-12.242, 5.45)
  line L8 (-12.242, 5.45) -> (0, 5.45)
  line L9 (0, 0) -> (0, 58.42) projected
  line L10 (0, 5.45) -> (0, 0)
  line L11 (-26.9178, 0) -> (-45.5, 0) projected
  line L12 (0, 0) -> (-26.9178, 0)
  line L13 (-26.9178, 0) -> (-25.4568, 1.87)
  point P0 (-43, 31.2191)
  dimension "d120" = 5.45
  constraints: 18 end point, 4 collinear, 2 perpendicular, 1 coincident, 1 horizontal, 1 parallel, 1 point on line
  measures "d120" distance between parallel lines of L12 L8
extrude "Выдавливание25" add sketch "Эскиз23" against normal blind 2
sketch "Эскиз24" plane through (-22.6372, -31.2191, -43) normal (1, 0, 0) x (0, 0, -1)
  line L0 (0, 0) -> (0, 58.42) projected
  line L1 (0, 10) -> (-8, 0)
  line L2 (0, 0) -> (-26.9178, 0) projected
  line L3 (-8, 0) -> (0, 0)
  line L4 (0, 10) -> (0, 0)
  point P0 (-43, 31.2191)
  dimension "d123" = 10
  dimension "d124" = 8
  constraints: 6 end point, 2 point on line, 1 collinear, 1 perpendicular
  measures "d123" distance from line of L2 L1.start
  measures "d124" distance of L1.end L0.start
extrude "Выдавливание26" cut sketch "Эскиз24" against normal blind 10
sketch "Эскиз25" plane through (24.1628, 27.2009, 0) normal (1, 0, 0) x (0, 0, -1)
  line L0 (21.4887, -51.5) -> (17.5432, -56.55) projected
  line L1 (19.5159, -54.025) -> (16.1211, -58.3702)
  line L2 (35, -58.42) -> (16.0822, -58.42) projected
  line L3 (16.0822, -58.42) -> (19.5199, -54.02) projected
  line L4 (16.0822, -58.42) -> (17.5432, -56.55) projected
  line L5 (16.0822, -58.42) -> (3.6598, -74.32)
  line L6 (3.6598, -74.32) -> (2.0837, -73.0887)
  line L7 (2.0837, -73.0887) -> (15.0052, -56.55)
  line L8 (15.0052, -56.55) -> (17.5432, -56.55)
  line L9 (27.9515, -43.228) -> (19.5199, -54.02) projected
  line L10 (18.5444, -52.02) -> (25.4135, -43.228) projected
  point P0 (0, -27.2009)
  dimension "d127" = 1.87
  dimension "d130" = 2
  dimension "d131" = 2
  dimension "d132" = 15.9
  constraints: 10 end point, 2 collinear, 2 perpendicular, 1 horizontal, 1 midpoint, 1 point on line
  measures "d127" distance between parallel lines of L2 L8
  measures "d130" distance between parallel lines of L9 L10
  measures "d131" distance between parallel lines of L5 L7
  measures "d132" distance from line of L2 L5.end
extrude "Выдавливание27" add sketch "Эскиз25" against normal up to surface (46.8 mm away)
sketch "Эскиз26" plane through (24.1628, -11.7991, -31.2548) normal (0, -0.6156615, -0.7880108) x (-1, 0, 0)
  line L0 (2, -15.8627) -> (2, -22.2713) projected
  ellipse E0 centre (12, -15.8627) end of major axis (12, -3.1725) minor radius 10 (12, -3.1725) -> (2, -15.8627) ccw projected
  line L1 (12, -3.1725) -> (25.16, -3.1725) projected
  line L2 (25.16, -0.8068) -> (25.16, -3.1725) projected
  line L3 (25.16, -0.8068) -> (46.8, -0.8068) projected
  line L4 (46.8, -0.8068) -> (48.18, -0.8068) projected
  line L5 (48.18, 17.1283) -> (48.18, -0.8068) projected
  line L6 (27, 17.1283) -> (48.18, 17.1283) projected
  line L7 (27, -0.315) -> (27, 17.1283) projected
  line L8 (25.16, -0.315) -> (27, -0.315) projected
  line L9 (25.16, 0) -> (25.16, -0.315) projected
  line L10 (0, 0) -> (25.16, 0) projected
  line L11 (0, 0.0234) -> (0, 0) projected
  line L12 (0, 0.0234) -> (-1.8, 0.0234) projected
  arc A0 (-1.8, 0.0234) -> (-5.3216, -2.0797) centre (-1.8, -3.9766) ccw projected
  line L13 (-5.3216, -2.0797) -> (-5.8, -5.3654) projected
  line L14 (-5.8, -5.3654) -> (-1.424, -19.0607) projected
  line L15 (0, -19.0607) -> (-1.424, -19.0607) projected
  line L16 (0, -44.8217) -> (0, -19.0607) projected
  line L17 (0, -44.8217) -> (46.8, -44.8217) projected
  line L18 (46.8, -24.6443) -> (46.8, -44.8217) projected
  line L19 (46.8, -24.6443) -> (46.8, -22.2713) projected
  line L20 (2, -22.2713) -> (46.8, -22.2713) construction
  circle A1 centre (-2.6539, -4.3253) radius 1.75 projected
  line L21 (46.8, -44.8217) -> (46.8, -26.2069) projected
  line L22 (2, -22.2713) -> (46.8, -22.2713) projected
  line L23 (46.8, -23.3703) -> (46.8, -22.2713)
  line L24 (0, -44.8217) -> (0, -19.0607) projected
  line L25 (0, -44.8217) -> (46.8, -44.8217) projected
  line L26 (0, -44.8217) -> (35.429, -44.8217)
  line L27 (0, -44.8217) -> (0, -26.2069)
  line L28 (0, -23.3703) -> (-1.424, -23.3703) projected
  arc A2 (41.8, -44.8217) -> (46.8, -39.8217) centre (41.8, -39.8217) ccw
  line L29 (0, -26.2069) -> (0, -44.8217)
  line L30 (0, -44.8217) -> (35.429, -44.8217)
  line L31 (46.8, -44.8217) -> (41.8, -44.8217)
  line L32 (35.429, -44.8217) -> (0, -44.8217)
  line L33 (46.8, -39.8217) -> (46.8, -44.8217)
  line L34 (0, -26.2069) -> (0, -36.0847) projected
  line L35 (0, -26.2069) -> (35.429, -44.8217)
  line L36 (46.8, -26.2069) -> (0, -26.2069) projected
  point P0 (24.1628, -9.9445)
  dimension "d135" = 5
  dimension "d138" = 0
  constraints: 18 end point, 7 collinear, 4 point on line, 3 tangent, 2 point on circle, 1 centre point, 1 perpendicular, 1 other
  measures "d135" radius of A2
  measures "d138" distance from line of L36 L27.end
extrude "Выдавливание28" cut sketch "Эскиз26" against normal blind 2 contours L18 L17 A2 | L35 L17 L16
fillet "Сопряжение4" radius 10 1 edges at (-11.2662, -46.5034, -2.8717)
sketch "Эскиз27" plane through (24.1628, -11.7991, -31.2548) normal (0, -0.6156615, -0.7880108) x (-1, 0, 0)
  circle A0 centre (42.4714, -40.6327) radius 1.75
  point P0 (24.1628, -9.9445)
  dimension "d140" = 3.5
  constraints: 1 centre point
  measures "d140" diameter of A0
extrude "Выдавливание29" cut sketch "Эскиз27" against normal blind 2
chamfer "Фаска1" distance 2 angle 45 1 edges at (25.9923, -25.8191, -12.5199)
sketch "Эскиз28" plane through (-22.6372, -31.2191, -13.5442) normal (0, 0.6156615, 0.7880108) x (1, 0, 0)
  circle A0 centre (4.3286, -14.4258) radius 1.75 projected
  arc A1 (8.9039, -18.6148) -> (13.555, -17.4673) centre (8.9039, -8.6148) ccw projected
  line L0 (13.555, -17.4673) -> (46.8, 0) projected
  line L1 (0, 0) -> (46.8, 0) projected
  line L2 (0, -13.6148) -> (0, 0) projected
  arc A2 (0, -13.6148) -> (5, -18.6148) centre (5, -13.6148) ccw projected
  line L3 (8.9039, -18.6148) -> (5, -18.6148) projected
  line L4 (8.9039, -18.6148) -> (8.9039, -10.4907)
  line L5 (8.9039, -10.4907) -> (0, -10.4907)
  line L6 (0, -13.6148) -> (0, 0) projected
  point P0 (22.6372, 16.2624)
  constraints: 4 end point, 1 perpendicular, 1 point on line, 1 vertical
extrude "Выдавливание30" add sketch "Эскиз28" along normal blind 2 contours L3 A2 L2 L5 L4
ref_plane "РабПлоскость1" through (3.1628, 27.2009, 0) normal (1, 0, 0) x (0, 0, -1)
sketch "Эскиз29" plane through (3.1628, 27.2009, 0) normal (1, 0, 0) x (0, 0, -1)
  line L0 (7.0854, -66.6868) -> (13.5442, -58.42) projected
  line L1 (13.5442, -58.42) -> (0.8352, -58.42)
  line L2 (0.8352, -58.42) -> (7.6153, -66.0086)
  line L3 (13.5442, -58.42) -> (7.6153, -66.0086)
  point P0 (0, -27.2009)
  constraints: 6 end point, 1 horizontal, 1 point on line
extrude "Выдавливание31" add sketch "Эскиз29" against normal blind 1.5
ref_plane "РабПлоскость2" through (-14.6372, -31.2191, -16.0822) normal (-1, 0, 0) x (0, 0, 1)
sketch "Эскиз30" plane through (-14.6372, -31.2191, -16.0822) normal (-1, 0, 0) x (0, 0, 1)
  line L0 (8.9968, -8.2668) -> (2.538, 0) projected
  line L1 (2.538, 0) -> (9.5729, -9.0042)
  line L2 (9.5729, -9.0042) -> (15.2403, 0)
  line L3 (-18.9178, 0) -> (18.5822, 0) projected
  line L4 (2.538, 0) -> (0.962, -1.2313) projected
  line L5 (15.2403, 0) -> (2.538, 0)
  point P0 (16.0822, 31.2191)
  constraints: 6 end point, 1 collinear, 1 horizontal, 1 point on line
extrude "Выдавливание32" add sketch "Эскиз30" against normal blind 1.5
ref_plane "РабПлоскость3" through (0, 0, -6) normal (0, 0, 1) x (1, 0, 0)
sketch "Эскиз31" plane through (0, 0, -6) normal (0, 0, 1) x (1, 0, 0)
  circle A0 centre (11.7328, -18.5923) radius 2.05 projected
  circle A1 centre (-11.7672, -18.5923) radius 2.05 projected
  circle A2 centre (11.7328, -18.5923) radius 1.5
  circle A3 centre (-11.7672, -18.5923) radius 1.5
  line L0 (-11.7672, -18.5923) -> (-11.7672, -29.3491) construction
  line L1 (-13.1372, -31.2191) -> (1.6628, -31.2191) projected
  line L2 (-11.7672, -29.3491) -> (11.7328, -29.3491)
  line L3 (22.1628, -29.3491) -> (-24.0172, -29.3491) projected
  line L4 (11.7328, -18.5923) -> (11.7328, -29.3491) construction
  line L5 (-15.2672, -18.5923) -> (-15.2672, -29.3491)
  line L6 (-8.2672, -18.5923) -> (-8.2672, -29.3491)
  line L7 (8.3547, -17.6766) -> (5.1907, -29.3491)
  line L8 (15.1109, -17.6766) -> (18.275, -29.3491)
  line L9 (-13.2672, -29.3491) -> (-10.2672, -29.3491)
  line L10 (-10.2672, -29.3491) -> (-10.2672, -21.7546)
  line L11 (-13.2672, -21.7546) -> (-13.2672, -29.3491)
  line L12 (9.4577, -21.252) -> (7.2629, -29.3491)
  line L13 (14.0079, -21.252) -> (16.2028, -29.3491)
  arc A4 (-13.2672, -21.7546) -> (-10.2672, -21.7546) centre (-11.7672, -18.5923) ccw
  arc A5 (-8.2672, -18.5923) -> (-15.2672, -18.5923) centre (-11.7672, -18.5923) ccw
  arc A6 (9.4577, -21.252) -> (14.0079, -21.252) centre (11.7328, -18.5923) ccw
  arc A7 (15.1109, -17.6766) -> (8.3547, -17.6766) centre (11.7328, -18.5923) ccw
  point P0 (0, 0)
  dimension "d155" = 3
  dimension "d156" = 3
  dimension "d159" = 2
  dimension "d160" = 2
  constraints: 24 end point, 8 point on circle, 6 centre point, 4 coincident, 3 parallel, 3 perpendicular, 2 tangent, 1 horizontal, 13 other
  measures "d155" diameter of A2
  measures "d156" diameter of A3
  measures "d159" distance between parallel lines of L12 L7
  measures "d160" distance between parallel lines of L5 L11
extrude "Выдавливание33" add sketch "Эскиз31" against normal blind 3.5 contours A0 | A1 | L10 A4 L11 L3 L5 A5 L6 L2 | L7 A7 L8 L3 L13 A6 L12 L2
sketch "Эскиз32" plane through (0, 0, -6) normal (0, 0, 1) x (1, 0, 0)
  circle A0 centre (-11.7672, -18.5923) radius 3.5 projected
  arc A1 (15.1109, -17.6766) -> (8.3547, -17.6766) centre (11.7328, -18.5923) ccw projected
  line L0 (24.1628, -11.7991) -> (-0.9972, -11.7991) projected
  arc A2 (9.4577, -21.252) -> (14.0079, -21.252) centre (11.7328, -18.5923) ccw projected
  circle A3 centre (-11.7672, -18.5923) radius 1.5 projected
  circle A4 centre (-11.7672, -18.5923) radius 1.5
  circle A5 centre (11.7328, -18.5923) radius 3.5
  circle A6 centre (11.7328, -18.5923) radius 1.5
  point P0 (0, 0)
  dimension "d163" = 3
  dimension "d164" = 3
  constraints: 3 centre point, 3 coincident, 1 concentric
  measures "d163" diameter of A4
  measures "d164" diameter of A6
extrude "Выдавливание34" add sketch "Эскиз32" along normal blind 2
sketch "Эскиз33" plane through (0, 0, 0) normal (0, 0, -1) x (-1, 0, 0)
  line L0 (-24.1628, 27.2009) -> (-13.8628, 27.2009) projected
  line L1 (-13.8628, 29.2009) -> (-13.8628, 27.2009) projected
  line L2 (-24.1628, 29.2009) -> (-13.8628, 29.2009) projected
  line L3 (-24.1628, 27.2009) -> (-24.1628, 29.2009) projected
  line L4 (16.0172, 27.2009) -> (26.0172, 27.2009) projected
  line L5 (26.0172, 27.2009) -> (26.0172, 29.2009) projected
  line L6 (26.0172, 29.2009) -> (16.0172, 29.2009) projected
  line L7 (16.0172, 29.2009) -> (16.0172, 27.2009) projected
  point P0 (0, 0)
extrude "Выдавливание35" add sketch "Эскиз33" along normal blind 0.5
sketch "Эскиз34" plane through (-26.0172, 27.2009, -43) normal (0, 1, 0) x (1, 0, 0)
  line L0 (6.5, -35.36) -> (6.5, -6.86) construction
  line L1 (5, -35.36) -> (5, -6.86)
  line L2 (8, -6.86) -> (8, -35.36)
  arc A0 (5, -35.36) -> (8, -35.36) centre (6.5, -35.36) ccw
  arc A1 (8, -6.86) -> (5, -6.86) centre (6.5, -6.86) ccw
  line L3 (0, 0) -> (50.18, 0) projected
  line L4 (0, -42.5) -> (0, 0) projected
  point P0 (26.0172, -43)
  point P1 (6.5, -21.11)
  dimension "d169" = 3
  dimension "d170" = 31.5
  dimension "d171" = 5.36
  dimension "d172" = 5
  constraints: 8 end point, 4 point on circle, 4 tangent, 2 centre point, 1 midpoint, 1 parallel, 1 vertical
  measures "d169" distance between parallel lines of L1 L2
  measures "d171" distance edge to line of A1 L3
  measures "d172" distance between parallel lines of L4 L1
extrude "Выдавливание36" cut sketch "Эскиз34" against normal blind 2
pattern_linear "Прямоуг.массив1" count 3 spacing 5.5 along (1, 0, 0) of "Выдавливание36"
sketch "Эскиз35" plane through (-26.0172, 26.6514, 2.8) normal (-1, 0, 0) x (0, 0, 1)
  line L0 (-36.83, -5.4404) -> (-8.43, -5.4404) construction
  line L1 (-36.83, -6.7404) -> (-8.43, -6.7404)
  line L2 (-8.43, -4.1404) -> (-36.83, -4.1404)
  arc A0 (-36.83, -4.1404) -> (-36.83, -6.7404) centre (-36.83, -5.4404) ccw
  arc A1 (-8.43, -6.7404) -> (-8.43, -4.1404) centre (-8.43, -5.4404) ccw
  line L3 (-45.8, -47.8704) -> (-45.8, 0.5496) projected
  line L4 (-3.3, 0.5496) -> (-45.8, 0.5496) projected
  point P0 (-2.8, -26.6514)
  point P1 (-22.63, -5.4404)
  dimension "d178" = 2.6
  dimension "d179" = 31
  dimension "d180" = 7.67
  dimension "d181" = 4.69
  constraints: 8 end point, 4 point on circle, 4 tangent, 2 centre point, 1 horizontal, 1 midpoint, 1 parallel
  measures "d178" distance between parallel lines of L1 L2
  measures "d180" distance edge to line of A0 L3
  measures "d181" distance between parallel lines of L4 L2
extrude "Выдавливание37" cut sketch "Эскиз35" against normal blind 2
pattern_linear "Прямоуг.массив2" count 4 spacing 6.2 along (0, -1, 0) of "Выдавливание37"
sketch "Эскиз36" plane through (-26.0172, 26.6514, 2.8) normal (-1, 0, 0) x (0, 0, 1)
  line L0 (-8.38, -40.9204) -> (-16.88, -40.9204)
  line L1 (-16.88, -40.9204) -> (-16.88, -47.1704)
  line L2 (-16.88, -47.1704) -> (-8.38, -47.1704)
  line L3 (-8.38, -47.1704) -> (-8.38, -40.9204)
  line L4 (-37.8, -57.8704) -> (-0.3, -57.8704) projected
  line L5 (-2.8, -3.4104) -> (-2.8, -56.0937) projected
  point P0 (-2.8, -26.6514)
  dimension "d187" = 10.7
  dimension "d188" = 5.58
  dimension "d189" = 6.25
  dimension "d190" = 8.5
  constraints: 8 end point, 2 parallel, 1 horizontal, 1 perpendicular
  measures "d187" distance between parallel lines of L4 L2
  measures "d188" distance between parallel lines of L5 L3
  measures "d189" distance between parallel lines of L0 L2
  measures "d190" distance between parallel lines of L1 L3
extrude "Выдавливание38" cut sketch "Эскиз36" against normal blind 2
sketch "Эскиз37" plane through (24.1628, -11.7991, -31.2548) normal (0, -0.6156615, -0.7880108) x (-1, 0, 0)
  circle A0 centre (-0.5286, -2.6327) radius 2.25 projected
  point P0 (24.1628, -9.9445)
sketch "Эскиз38" plane through (24.1628, -11.7991, -31.2548) normal (0, -0.6156615, -0.7880108) x (-1, 0, 0)
  circle A0 centre (-2.6539, -4.3253) radius 1.75 projected
  point P0 (24.1628, -9.9445)
extrude "Выдавливание39" add sketch "Эскиз38" against normal up to surface (2 mm away)
extrude "Выдавливание40" cut sketch "Эскиз37" against normal blind 4
